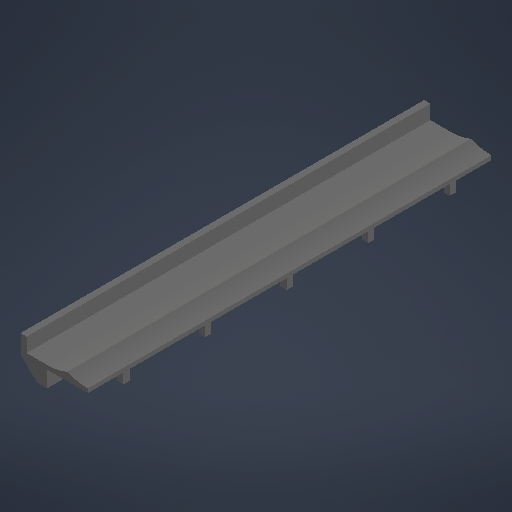
# Autodesk Inventor part: front_rail
Saved by Autodesk Inventor 2026 (Build 300175050, 175E)
## iProperties
Created: 2025-09-28
Part Number: front_rail
Material: 一般
Document SubType Name: Modeling
Designer: hibik
Density: 1 g/cm^3
Appearance: 既定
Author: hibik
Autodesk Inventor part; units mm, degrees
ref_plane "YZ Plane" through (0, 0, 0) normal (1, 0, 0) x (0, 1, 0)
ref_plane "XZ Plane" through (0, 0, 0) normal (0, 1, 0) x (-1, 0, 0)
ref_plane "XY Plane" through (0, 0, 0) normal (0, 0, 1) x (1, 0, 0)
sketch "スケッチ1" plane through (0, 0, 0) normal (0, 1, 0) x (-1, 0, 0)
  line L0 (0, 99) -> (20, 99)
  line L1 (20, 99) -> (20, -99)
  line L2 (20, -99) -> (0, -99)
  line L3 (0, -99) -> (0, 99)
  line L4 (20, -99) -> (20, -109)
  line L5 (20, -109) -> (9, -109)
  line L6 (9, -109) -> (11, -99)
  line L7 (10.5, 99) -> (8.5, 88.5)
  line L8 (8.5, 88.5) -> (20, 88.5)
  point P0 (0, 0)
  point P1 (0, 0)
  point P2 (10, -99)
  point P3 (10, 99)
  dimension "d0" = 198
  dimension "d1" = 20
  dimension "d4" = 10
  dimension "d5" = 1
  dimension "d6" = 1
  dimension "d7" = 10.5
  dimension "d8" = 1.5
  dimension "d9" = 0.5
  constraints: 18 end point, 3 midpoint, 3 perpendicular, 3 point on line, 2 parallel, 1 coincident, 1 horizontal, 1 vertical
  measures "d0" distance of L0.end L1.end
  measures "d1" distance of L0.start L0.end
  measures "d4" distance of L1.end L4.end
  measures "d5" distance of point (10, -99) L6.end
  measures "d6" horizontal distance of point (10, -99) L5.end
  measures "d7" distance between parallel lines of L0 L8
  measures "d8" horizontal distance of point (10, 99) L7.end
  measures "d9" distance of point (10, 99) L7.start
extrude "押し出し1" add sketch "スケッチ1" along normal blind 5.5 contours L0 L7 L8 L1 L2 L3 | L2 L4 L5 L6
sketch "スケッチ2" plane through (0, 5.5, 0) normal (0, 1, 0) x (1, 0, 0)
  line L0 (-20, 109) -> (-20, -88.5) projected
  line L1 (-20, -1.5) -> (-17, -1.5)
  line L2 (-17, -1.5) -> (-17, 1.5)
  line L3 (-17, 1.5) -> (-20, 1.5)
  line L4 (-20, 1.5) -> (-20, -1.5)
  line L5 (0, -99) -> (0, 99) projected
  line L6 (0, -1.5) -> (-3, -1.5)
  line L7 (-3, -1.5) -> (-3, 1.5)
  line L8 (-3, 1.5) -> (0, 1.5)
  line L9 (0, 1.5) -> (0, -1.5)
  point P0 (0, 0)
  point P1 (-17, 0)
  point P2 (0, 0)
  point P3 (0, 1.5)
  dimension "d10" = 3
  dimension "d11" = 3
  constraints: 16 end point, 4 parallel, 4 point on line, 2 horizontal, 2 midpoint, 2 perpendicular, 1 collinear, 1 horizontal alignment
  measures "d10" distance of L1.start L1.end
  measures "d11" distance of L1.end L2.end
extrude "押し出し2" cut sketch "スケッチ2" against normal through all
pattern_linear "矩形状パターン1" count 3 spacing 40 along (0, 0, -1) count 3 spacing 40 along (0, 0, 1) of "押し出し2"
sketch "スケッチ3" plane through (0, 5.5, 0) normal (0, 1, 0) x (1, 0, 0)
  line L0 (-20, -88.5) -> (-8.5, -88.5) projected
  line L1 (-20, -99) -> (0, -99)
  line L2 (0, -99) -> (0, 99)
  line L3 (-20, 109) -> (-20, -88.4991)
  line L4 (-20, -38.5) -> (-17, -38.5) projected
  line L5 (-17, -38.5) -> (-17, -41.5) projected
  line L6 (-17, -41.5) -> (-20, -41.5) projected
  line L7 (-20, -41.5) -> (-20, -78.5) projected
  line L8 (-20, -78.5) -> (-17, -78.5) projected
  line L9 (-17, -78.5) -> (-17, -81.5) projected
  line L10 (-17, -81.5) -> (-20, -81.5) projected
  line L11 (-20, -81.5) -> (-20, -88.5) projected
  line L12 (-20, -88.5) -> (-8.5, -88.5) projected
  line L13 (-8.5, -88.5) -> (-10.5, -99)
  line L14 (-10.5, -99) -> (0, -99) projected
  line L15 (0, -99) -> (0, -81.5) projected
  line L16 (0, -81.5) -> (-3, -81.5) projected
  line L17 (-3, -81.5) -> (-3, -78.5) projected
  line L18 (-3, -78.5) -> (0, -78.5) projected
  line L19 (0, -78.5) -> (0, -41.5) projected
  line L20 (0, -41.5) -> (-3, -41.5) projected
  line L21 (-3, -41.5) -> (-3, -38.5) projected
  line L22 (-3, -38.5) -> (0, -38.5) projected
  line L23 (0, -38.5) -> (0, -1.5) projected
  line L24 (0, -1.5) -> (-3, -1.5) projected
  line L25 (-3, -1.5) -> (-3, 1.5) projected
  line L26 (-3, 1.5) -> (0, 1.5) projected
  line L27 (0, 1.5) -> (0, 38.5) projected
  line L28 (0, 38.5) -> (-3, 38.5) projected
  line L29 (-3, 38.5) -> (-3, 41.5) projected
  line L30 (-3, 41.5) -> (0, 41.5) projected
  line L31 (0, 41.5) -> (0, 78.5) projected
  line L32 (0, 78.5) -> (-3, 78.5) projected
  line L33 (-3, 78.5) -> (-3, 81.5) projected
  line L34 (-3, 81.5) -> (0, 81.5) projected
  line L35 (0, 81.5) -> (0, 99) projected
  line L36 (-9, 109) -> (-20, 109) projected
  line L37 (-20, 109) -> (-20, 81.5) projected
  line L38 (-20, 81.5) -> (-17, 81.5) projected
  line L39 (-17, 81.5) -> (-17, 78.5) projected
  line L40 (-17, 78.5) -> (-20, 78.5) projected
  line L41 (-20, 78.5) -> (-20, 41.5) projected
  line L42 (-20, 41.5) -> (-17, 41.5) projected
  line L43 (-17, 41.5) -> (-17, 38.5) projected
  line L44 (-17, 38.5) -> (-20, 38.5) projected
  line L45 (-20, 38.5) -> (-20, 1.5) projected
  line L46 (-20, 1.5) -> (-17, 1.5) projected
  line L47 (-17, 1.5) -> (-17, -1.5) projected
  line L48 (-17, -1.5) -> (-20, -1.5) projected
  line L49 (-20, -1.5) -> (-20, -38.5) projected
  line L50 (-20, 109) -> (-20, 81.5) projected
  line L51 (-20, -99) -> (-20, -88.4991)
  line L52 (-9, 109) -> (0, 109)
  line L53 (0, 99) -> (0, 109)
  line L54 (0, 99) -> (-20, 99)
  point P0 (0, 0)
  point P1 (-11, 99)
  point P2 (0, -78.5)
  point P3 (0, -38.5)
  point P4 (0, 41.5)
  point P5 (0, 81.5)
  point P6 (-20, -88.4991)
  constraints: 16 end point, 3 point on line, 2 horizontal, 2 perpendicular, 2 vertical, 1 parallel
extrude "押し出し3" cut sketch "スケッチ3" against normal through all contours L3 L10 L9 L8 L6 L5 L4 L48 L47 L46 L44 L43 L42 L40 L39 L38 L54 L2 L34 L33 L32 L30 L29 L28 L26 L25 L24 L22 L21 L20 L18 L17 L16 L1 L13 L0 | L3 L8 L9 L10 | L3 L4 L5 L6 | L16 L17 L18 L2 | L3 L46 L47 L48 | L20 L21 L22 L2 | L3 L42 L43 L44 | L24 L25 L26 L2 | L3 L38 L39 L40 | L28 L29 L30 L2 | L3 L36 L52 L53 L54 | L32 L33 L34 L2
extrude "押し出し4" add sketch "スケッチ3" against normal blind 5 contours L3 L8 L9 L10 | L3 L4 L5 L6 | L16 L17 L18 L2 | L3 L46 L47 L48 | L20 L21 L22 L2 | L3 L42 L43 L44 | L24 L25 L26 L2 | L3 L38 L39 L40 | L28 L29 L30 L2 | L32 L33 L34 L2
extrude "押し出し5" add sketch "スケッチ3" along normal blind 2 contours L3 L10 L9 L8 L6 L5 L4 L48 L47 L46 L44 L43 L42 L40 L39 L38 L54 L2 L34 L33 L32 L30 L29 L28 L26 L25 L24 L22 L21 L20 L18 L17 L16 L1 L13 L0 | L0 L13 L1 L51 | L3 L8 L9 L10 | L3 L4 L5 L6 | L16 L17 L18 L2 | L3 L46 L47 L48 | L20 L21 L22 L2 | L3 L42 L43 L44 | L24 L25 L26 L2 | L3 L38 L39 L40 | L28 L29 L30 L2 | L32 L33 L34 L2
sketch "スケッチ4" plane through (-20, 5.5, 99) normal (0, 0, 1) x (1, 0, 0)
  arc A0 (0, 2) -> (10, 4) centre (0, 28) ccw
  line L0 (0, 2) -> (20, 2)
  arc A1 (10, 4) -> (20, 2) centre (20, 28) ccw
  line L1 (10, 4) -> (10, 2) construction
  point P0 (20, -5.5)
  point P1 (14.6904, 2)
  point P2 (5.3096, 2)
  dimension "d27" = 2
  constraints: 4 end point, 4 point on circle, 2 centre point, 1 midpoint
  measures "d27" distance of L1.start L1.end
extrude "押し出し6" add sketch "スケッチ4" against normal up to surface (198 mm away)
sketch "スケッチ8" plane through (-20, 5.5, 99) normal (0, 0, 1) x (1, 0, 0)
  arc A0 (0, 2) -> (10, 4) centre (0, 28) ccw projected
  line L0 (0, 2) -> (-10, 2)
  line L1 (-10, 2) -> (-10, -8)
  line L2 (-10, -8) -> (0, -8)
  line L3 (0, -8) -> (0, 2)
  line L4 (-10, -8) -> (-13, -8)
  line L5 (-13, -8) -> (-13, 9)
  line L6 (-13, 9) -> (-10, 9)
  line L7 (-10, 9) -> (-10, -8)
  point P0 (20, -5.5)
  dimension "d44" = 7
  dimension "d45" = 3
  dimension "d46" = 10
  dimension "d47" = 10
  constraints: 16 end point, 4 parallel, 2 horizontal, 2 perpendicular
  measures "d44" distance between parallel lines of L6 L0
  measures "d45" distance of L1.end L4.end
  measures "d46" distance of L1.end L2.end
  measures "d47" distance of L2.end L0.start
extrude "押し出し9" add sketch "スケッチ8" against normal up to surface (198 mm away)
chamfer "面取り3" distance 8 angle 45 1 edges at (-33, -2.5, 0)
